Autodesk Inventor part; units mm, degrees
(part 2 of 4)
  arc A605 (9.3443, -15.2712) -> (9.707, -15.104) centre (0.9435, 3.4284) ccw
  arc A606 (10.7855, -14.5545) -> (11.1341, -14.3593) centre (0.9435, 3.4284) ccw
  arc A607 (12.1661, -13.7268) -> (12.4983, -13.5049) centre (0.9435, 3.4284) ccw
  arc A608 (13.4775, -12.7935) -> (13.7912, -12.5461) centre (0.9435, 3.4284) ccw
  arc A609 (14.7116, -11.76) -> (15.005, -11.4889) centre (0.9435, 3.4284) ccw
  arc A610 (15.8608, -10.633) -> (16.132, -10.3397) centre (0.9435, 3.4284) ccw
  arc A611 (16.9181, -9.4192) -> (17.1654, -9.1055) centre (0.9435, 3.4284) ccw
  arc A612 (17.8769, -8.1263) -> (18.0988, -7.7941) centre (0.9435, 3.4284) ccw
  arc A613 (18.7313, -6.7621) -> (18.9264, -6.4136) centre (0.9435, 3.4284) ccw
  arc A614 (19.476, -5.3351) -> (19.6432, -4.9723) centre (0.9435, 3.4284) ccw
  arc A615 (20.1064, -3.854) -> (20.2447, -3.4792) centre (0.9435, 3.4284) ccw
  arc A616 (20.6187, -2.3281) -> (20.7271, -1.9436) centre (0.9435, 3.4284) ccw
  arc A617 (21.0097, -0.7666) -> (21.0876, -0.3748) centre (0.9435, 3.4284) ccw
  arc A618 (21.277, 0.8207) -> (21.3239, 1.2174) centre (0.9435, 3.4284) ccw
  arc A619 (21.4189, 2.4241) -> (21.4346, 2.8232) centre (0.9435, 3.4284) ccw
  arc A620 (21.4346, 4.0336) -> (21.4189, 4.4328) centre (0.9435, 3.4284) ccw
  arc A621 (21.3239, 5.6395) -> (21.277, 6.0362) centre (0.9435, 3.4284) ccw
  arc A622 (21.0876, 7.2317) -> (21.0097, 7.6235) centre (0.9435, 3.4284) ccw
  arc A623 (20.7271, 8.8005) -> (20.6187, 9.1849) centre (0.9435, 3.4284) ccw
  arc A624 (20.2447, 10.3361) -> (20.1064, 10.7109) centre (0.9435, 3.4284) ccw
  arc A625 (19.6432, 11.8292) -> (19.476, 12.1919) centre (0.9435, 3.4284) ccw
  arc A626 (18.9264, 13.2704) -> (18.7313, 13.619) centre (0.9435, 3.4284) ccw
  arc A627 (18.0988, 14.651) -> (17.8769, 14.9832) centre (0.9435, 3.4284) ccw
  arc A628 (17.1654, 15.9624) -> (16.9181, 16.2761) centre (0.9435, 3.4284) ccw
  arc A629 (16.132, 17.1965) -> (15.8608, 17.4899) centre (0.9435, 3.4284) ccw
  arc A630 (15.005, 18.3458) -> (14.7116, 18.6169) centre (0.9435, 3.4284) ccw
  arc A631 (13.7912, 19.403) -> (13.4775, 19.6503) centre (0.9435, 3.4284) ccw
  arc A632 (12.4983, 20.3618) -> (12.1661, 20.5837) centre (0.9435, 3.4284) ccw
  arc A633 (11.1341, 21.2162) -> (10.7855, 21.4113) centre (0.9435, 3.4284) ccw
  arc A634 (9.707, 21.9609) -> (9.3443, 22.1281) centre (0.9435, 3.4284) ccw
  arc A635 (8.226, 22.5913) -> (7.8512, 22.7296) centre (0.9435, 3.4284) ccw
  arc A636 (6.7, 23.1036) -> (6.3156, 23.212) centre (0.9435, 3.4284) ccw
  arc A637 (5.1386, 23.4946) -> (4.7468, 23.5725) centre (0.9435, 3.4284) ccw
  arc A638 (3.5513, 23.7619) -> (3.1546, 23.8088) centre (0.9435, 3.4284) ccw
  arc A639 (1.9479, 23.9038) -> (1.5487, 23.9195) centre (0.9435, 3.4284) ccw
  line L0 (-21.5565, 3.4284) -> (23.4435, 3.4284)
  line L1 (0.9435, -19.0716) -> (0.9435, 25.9284)
  point P0 (0, 0)
  constraints: 960 point on circle, 480 centre point, 4 end point, 2 horizontal alignment, 2 vertical alignment, 476 other
extrude "押し出し1" add sketch "スケッチ1" along normal blind 3
sketch "スケッチ2" plane through (0, 0, 3) normal (0, 0, 1) x (1, 0, 0)
  arc A0 (1.2215, 23.1029) -> (1.1332, 22.8025) centre (6.2327, 21.4655) ccw projected
  arc A1 (1.1332, 22.8025) -> (0.7539, 22.8025) centre (0.9435, 3.4284) ccw projected
  arc A2 (0.7539, 22.8025) -> (0.6655, 23.1029) centre (-4.3457, 21.4655) ccw projected
  arc A3 (0.6655, 23.1029) -> (0.5317, 23.4735) centre (-5.4255, 21.1133) ccw projected
  arc A4 (0.5317, 23.4735) -> (0.3383, 23.9195) centre (-6.5223, 20.6793) ccw projected
  arc A5 (0.3383, 23.9195) -> (-0.0608, 23.9038) centre (0.9435, 3.4284) ccw projected
  arc A6 (-0.0608, 23.9038) -> (-0.2187, 23.444) centre (7.0329, 21.2118) ccw projected
  arc A7 (-0.2187, 23.444) -> (-0.323, 23.0641) centre (5.9054, 21.5585) ccw projected
  arc A8 (-0.323, 23.0641) -> (-0.3875, 22.7577) centre (4.8013, 21.8249) ccw projected
  arc A9 (-0.3875, 22.7577) -> (-0.7656, 22.7279) centre (0.9435, 3.4284) ccw projected
  arc A10 (-0.7656, 22.7279) -> (-0.8773, 23.0205) centre (-5.7445, 20.995) ccw projected
  arc A11 (-0.8773, 23.0205) -> (-1.0397, 23.3794) centre (-6.7934, 20.5591) ccw projected
  arc A12 (-1.0397, 23.3794) -> (-1.2675, 23.8088) centre (-7.8528, 20.0403) ccw projected
  arc A13 (-1.2675, 23.8088) -> (-1.6642, 23.7619) centre (0.9435, 3.4284) ccw projected
  arc A14 (-1.6642, 23.7619) -> (-1.7855, 23.2911) centre (5.6188, 21.6348) ccw projected
  arc A15 (-1.7855, 23.2911) -> (-1.8597, 22.9042) centre (4.4676, 21.8919) ccw projected
  arc A16 (-1.8597, 22.9042) -> (-1.9, 22.5936) centre (3.346, 22.0709) ccw projected
  arc A17 (-1.9, 22.5936) -> (-2.2745, 22.5343) centre (0.9435, 3.4284) ccw projected
  arc A18 (-2.2745, 22.5343) -> (-2.4088, 22.8172) centre (-7.1022, 20.4161) ccw projected
  arc A19 (-2.4088, 22.8172) -> (-2.5989, 23.1623) centre (-8.1136, 19.8993) ccw projected
  arc A20 (-2.5989, 23.1623) -> (-2.8597, 23.5725) centre (-9.129, 19.299) ccw projected
  arc A21 (-2.8597, 23.5725) -> (-3.2515, 23.4946) centre (0.9435, 3.4284) ccw projected
  arc A22 (-3.2515, 23.4946) -> (-3.3355, 23.0158) centre (4.176, 21.9455) ccw projected
  arc A23 (-3.3355, 23.0158) -> (-3.3791, 22.6242) centre (3.0081, 22.1115) ccw projected
  arc A24 (-3.3791, 22.6242) -> (-3.3949, 22.3115) centre (1.8759, 22.2019) ccw projected
  arc A25 (-3.3949, 22.3115) -> (-3.7636, 22.2229) centre (0.9435, 3.4284) ccw projected
  arc A26 (-3.7636, 22.2229) -> (-3.9197, 22.4944) centre (-8.4102, 19.7324) ccw projected
  arc A27 (-3.9197, 22.4944) -> (-4.1363, 22.8235) centre (-9.378, 19.1379) ccw projected
  arc A28 (-4.1363, 22.8235) -> (-4.4285, 23.212) centre (-10.3432, 18.4597) ccw projected
  arc A29 (-4.4285, 23.212) -> (-4.813, 23.1036) centre (0.9435, 3.4284) ccw projected
  arc A30 (-4.813, 23.1036) -> (-4.8591, 22.6197) centre (2.7132, 22.142) ccw projected
  arc A31 (-4.8591, 22.6197) -> (-4.8718, 22.2259) centre (1.5359, 22.2159) ccw projected
  arc A32 (-4.8718, 22.2259) -> (-4.863, 21.9129) centre (0.4001, 22.2172) ccw projected
  arc A33 (-4.863, 21.9129) -> (-5.2237, 21.7957) centre (0.9435, 3.4284) ccw projected
  arc A34 (-5.2237, 21.7957) -> (-5.4006, 22.0541) centre (-9.6606, 18.9483) ccw projected
  arc A35 (-5.4006, 22.0541) -> (-5.6424, 22.3652) centre (-10.5787, 18.2796) ccw projected
  arc A36 (-5.6424, 22.3652) -> (-5.9641, 22.7296) centre (-11.4877, 17.5279) ccw projected
  arc A37 (-5.9641, 22.7296) -> (-6.3389, 22.5913) centre (0.9435, 3.4284) ccw projected
  arc A38 (-6.3389, 22.5913) -> (-6.3469, 22.1053) centre (1.2395, 22.2232) ccw projected
  arc A39 (-6.3469, 22.1053) -> (-6.3287, 21.7117) centre (0.06, 22.2045) ccw projected
  arc A40 (-6.3287, 21.7117) -> (-6.2954, 21.4003) centre (-1.0724, 22.1166) ccw projected
  arc A41 (-6.2954, 21.4003) -> (-6.6458, 21.2552) centre (0.9435, 3.4284) ccw projected
  arc A42 (-6.6458, 21.2552) -> (-6.8424, 21.4989) centre (-10.8456, 18.0685) ccw projected
  arc A43 (-6.8424, 21.4989) -> (-7.1078, 21.7901) centre (-11.7084, 17.3298) ccw projected
  arc A44 (-7.1078, 21.7901) -> (-7.4572, 22.1281) centre (-12.5556, 16.5091) ccw projected
  arc A45 (-7.4572, 22.1281) -> (-7.82, 21.9609) centre (0.9435, 3.4284) ccw projected
  arc A46 (-7.82, 21.9609) -> (-7.7898, 21.4757) centre (-0.2361, 22.1885) ccw projected
  arc A47 (-7.7898, 21.4757) -> (-7.7408, 21.0848) centre (-1.4104, 22.0773) ccw projected
  arc A48 (-7.7408, 21.0848) -> (-7.6832, 20.7769) centre (-2.5324, 21.9009) ccw projected
  arc A49 (-7.6832, 20.7769) -> (-8.0211, 20.6048) centre (0.9435, 3.4284) ccw projected
  arc A50 (-8.0211, 20.6048) -> (-8.2362, 20.8323) centre (-11.9579, 17.0984) ccw projected
  arc A51 (-8.2362, 20.8323) -> (-8.5237, 21.1018) centre (-12.7601, 16.2943) ccw projected
  arc A52 (-8.5237, 21.1018) -> (-8.8985, 21.4113) centre (-13.5403, 15.4096) ccw projected
  arc A53 (-8.8985, 21.4113) -> (-9.247, 21.2162) centre (0.9435, 3.4284) ccw projected
  arc A54 (-9.247, 21.2162) -> (-9.1789, 20.7348) centre (-1.7043, 22.0381) ccw projected
  arc A55 (-9.1789, 20.7348) -> (-9.0993, 20.349) centre (-2.8663, 21.8351) ccw projected
  arc A56 (-9.0993, 20.349) -> (-9.0177, 20.0466) centre (-3.971, 21.5712) ccw projected
  arc A57 (-9.0177, 20.0466) -> (-9.3411, 19.8485) centre (0.9435, 3.4284) ccw projected
  arc A58 (-9.3411, 19.8485) -> (-9.5734, 20.0585) centre (-12.9906, 16.044) ccw projected
  arc A59 (-9.5734, 20.0585) -> (-9.8811, 20.3045) centre (-13.7273, 15.1795) ccw projected
  arc A60 (-9.8811, 20.3045) -> (-10.279, 20.5837) centre (-14.4357, 14.2363) ccw projected
  arc A61 (-10.279, 20.5837) -> (-10.6112, 20.3618) centre (0.9435, 3.4284) ccw projected
  arc A62 (-10.6112, 20.3618) -> (-10.5055, 19.8873) centre (-3.1562, 21.773) ccw projected
  arc A63 (-10.5055, 19.8873) -> (-10.3959, 19.5089) centre (-4.2988, 21.4794) ccw projected
  arc A64 (-10.3959, 19.5089) -> (-10.2909, 19.2138) centre (-5.3794, 21.1297) ccw projected
  arc A65 (-10.2909, 19.2138) -> (-10.5977, 18.9909) centre (0.9435, 3.4284) ccw projected
  arc A66 (-10.5977, 18.9909) -> (-10.8458, 19.182) centre (-13.9375, 14.9118) ccw projected
  arc A67 (-10.8458, 19.182) -> (-11.1718, 19.4032) centre (-14.604, 13.9922) ccw projected
  arc A68 (-11.1718, 19.4032) -> (-11.5904, 19.6503) centre (-15.2362, 12.9963) ccw projected
  arc A69 (-11.5904, 19.6503) -> (-11.9041, 19.403) centre (0.9435, 3.4284) ccw projected
  arc A70 (-11.9041, 19.403) -> (-11.7616, 18.9383) centre (-4.5829, 21.3947) ccw projected
  arc A71 (-11.7616, 18.9383) -> (-11.6226, 18.5696) centre (-5.6989, 21.0125) ccw projected
  arc A72 (-11.6226, 18.5696) -> (-11.4947, 18.2837) centre (-6.7487, 20.579) ccw projected
  arc A73 (-11.4947, 18.2837) -> (-11.7831, 18.0374) centre (0.9435, 3.4284) ccw projected
  arc A74 (-11.7831, 18.0374) -> (-12.0454, 18.2085) centre (-14.7926, 13.7089) ccw projected
  arc A75 (-12.0454, 18.2085) -> (-12.3878, 18.4034) centre (-15.3849, 12.7398) ccw projected
  arc A76 (-12.3878, 18.4034) -> (-12.8246, 18.6169) centre (-15.9371, 11.6974) ccw projected
  arc A77 (-12.8246, 18.6169) -> (-13.1179, 18.3458) centre (0.9435, 3.4284) ccw projected
  arc A78 (-13.1179, 18.3458) -> (-12.9393, 17.8936) centre (-5.9755, 20.9058) ccw projected
  arc A79 (-12.9393, 17.8936) -> (-12.7719, 17.537) centre (-7.058, 20.4371) ccw projected
  arc A80 (-12.7719, 17.537) -> (-12.6219, 17.2621) centre (-8.0706, 19.9226) ccw projected
  arc A81 (-12.6219, 17.2621) -> (-12.8901, 16.9939) centre (0.9435, 3.4284) ccw projected
  arc A82 (-12.8901, 16.9939) -> (-13.165, 17.1438) centre (-15.5507, 12.4426) ccw projected
  arc A83 (-13.165, 17.1438) -> (-13.5217, 17.3113) centre (-16.0652, 11.43) ccw projected
  arc A84 (-13.5217, 17.3113) -> (-13.9738, 17.4899) centre (-16.5338, 10.3475) ccw projected
  arc A85 (-13.9738, 17.4899) -> (-14.2449, 17.1965) centre (0.9435, 3.4284) ccw projected
  arc A86 (-14.2449, 17.1965) -> (-14.0314, 16.7598) centre (-7.3254, 20.309) ccw projected
  arc A87 (-14.0314, 16.7598) -> (-13.8365, 16.4174) centre (-8.3678, 19.7569) ccw projected
  arc A88 (-13.8365, 16.4174) -> (-13.6655, 16.1551) centre (-9.3369, 19.1645) ccw projected
  arc A89 (-13.6655, 16.1551) -> (-13.9118, 15.8667) centre (0.9435, 3.4284) ccw projected
  arc A90 (-13.9118, 15.8667) -> (-14.1976, 15.9946) centre (-16.2071, 11.1207) ccw projected
  arc A91 (-14.1976, 15.9946) -> (-14.5663, 16.1335) centre (-16.6405, 10.0708) ccw projected
  arc A92 (-14.5663, 16.1335) -> (-15.0311, 16.2761) centre (-17.0228, 8.9549) ccw projected
  arc A93 (-15.0311, 16.2761) -> (-15.2784, 15.9624) centre (0.9435, 3.4284) ccw projected
  arc A94 (-15.2784, 15.9624) -> (-15.0312, 15.5438) centre (-8.6244, 19.6082) ccw projected
  arc A95 (-15.0312, 15.5438) -> (-14.8101, 15.2177) centre (-9.6202, 18.976) ccw projected
  arc A96 (-14.8101, 15.2177) -> (-14.619, 14.9696) centre (-10.5399, 18.3094) ccw projected
  arc A97 (-14.619, 14.9696) -> (-14.8419, 14.6628) centre (0.9435, 3.4284) ccw projected
  arc A98 (-14.8419, 14.6628) -> (-15.1369, 14.7679) centre (-16.7577, 9.7513) ccw projected
  arc A99 (-15.1369, 14.7679) -> (-15.5153, 14.8775) centre (-17.1075, 8.6707) ccw projected
  arc A100 (-15.5153, 14.8775) -> (-15.9898, 14.9832) centre (-17.401, 7.5282) ccw projected
  arc A101 (-15.9898, 14.9832) -> (-16.2118, 14.651) centre (0.9435, 3.4284) ccw projected
  arc A102 (-16.2118, 14.651) -> (-15.9326, 14.2531) centre (-9.8643, 18.8076) ccw projected
  arc A103 (-15.9326, 14.2531) -> (-15.6865, 13.9454) centre (-10.8075, 18.0992) ccw projected
  arc A104 (-15.6865, 13.9454) -> (-15.4765, 13.713) centre (-11.672, 17.3626) ccw projected
  arc A105 (-15.4765, 13.713) -> (-15.6747, 13.3897) centre (0.9435, 3.4284) ccw projected
  arc A106 (-15.6747, 13.3897) -> (-15.977, 13.4713) centre (-17.1992, 8.343) ccw projected
  arc A107 (-15.977, 13.4713) -> (-16.3629, 13.5508) centre (-17.4631, 7.2383) ccw projected
  arc A108 (-16.3629, 13.5508) -> (-16.8442, 13.619) centre (-17.6661, 6.0763) ccw projected
  arc A109 (-16.8442, 13.619) -> (-17.0394, 13.2704) centre (0.9435, 3.4284) ccw projected
  arc A110 (-17.0394, 13.2704) -> (-16.7298, 12.8956) centre (-11.0376, 17.9123) ccw projected
  arc A111 (-16.7298, 12.8956) -> (-16.4604, 12.6082) centre (-11.9224, 17.132) ccw projected
  arc A112 (-16.4604, 12.6082) -> (-16.2328, 12.393) centre (-12.7264, 16.3298) ccw projected
  arc A113 (-16.2328, 12.393) -> (-16.405, 12.0551) centre (0.9435, 3.4284) ccw projected
  arc A114 (-16.405, 12.0551) -> (-16.7128, 12.1128) centre (-17.5289, 6.9044) ccw projected
  arc A115 (-16.7128, 12.1128) -> (-17.1037, 12.1618) centre (-17.7053, 5.7824) ccw projected
  arc A116 (-17.1037, 12.1618) -> (-17.5889, 12.1919) centre (-17.8165, 4.608) ccw projected
  arc A117 (-17.5889, 12.1919) -> (-17.7561, 11.8292) centre (0.9435, 3.4284) ccw projected
  arc A118 (-17.7561, 11.8292) -> (-17.4181, 11.4798) centre (-12.1371, 16.9276) ccw projected
  arc A119 (-17.4181, 11.4798) -> (-17.127, 11.2144) centre (-12.9579, 16.0804) ccw projected
  arc A120 (-17.127, 11.2144) -> (-16.8832, 11.0178) centre (-13.6965, 15.2175) ccw projected
  arc A121 (-16.8832, 11.0178) -> (-17.0283, 10.6674) centre (0.9435, 3.4284) ccw projected
  arc A122 (-17.0283, 10.6674) -> (-17.3397, 10.7007) centre (-17.7447, 5.4443) ccw projected
  arc A123 (-17.3397, 10.7007) -> (-17.7333, 10.7189) centre (-17.8325, 4.312) ccw projected
  arc A124 (-17.7333, 10.7189) -> (-18.2193, 10.7109) centre (-17.8512, 3.1325) ccw projected
  arc A125 (-18.2193, 10.7109) -> (-18.3576, 10.3361) centre (0.9435, 3.4284) ccw projected
  arc A126 (-18.3576, 10.3361) -> (-17.9932, 10.0143) centre (-13.1559, 15.8597) ccw projected
  arc A127 (-17.9932, 10.0143) -> (-17.6821, 9.7726) centre (-13.9077, 14.9507) ccw projected
  arc A128 (-17.6821, 9.7726) -> (-17.4237, 9.5957) centre (-14.5763, 14.0325) ccw projected
  arc A129 (-17.4237, 9.5957) -> (-17.5409, 9.235) centre (0.9435, 3.4284) ccw projected
  arc A130 (-17.5409, 9.235) -> (-17.8539, 9.2438) centre (-17.8452, 3.9719) ccw projected
  arc A131 (-17.8539, 9.2438) -> (-18.2477, 9.2311) centre (-17.8439, 2.8361) ccw projected
  arc A132 (-18.2477, 9.2311) -> (-18.7317, 9.1849) centre (-17.7701, 1.6588) ccw projected
  arc A133 (-18.7317, 9.1849) -> (-18.8401, 8.8005) centre (0.9435, 3.4284) ccw projected
  arc A134 (-18.8401, 8.8005) -> (-18.4516, 8.5083) centre (-14.0878, 14.7151) ccw projected
  arc A135 (-18.4516, 8.5083) -> (-18.1225, 8.2917) centre (-14.7659, 13.7499) ccw projected
  arc A136 (-18.1225, 8.2917) -> (-17.851, 8.1356) centre (-15.3605, 12.7822) ccw projected
  arc A137 (-17.851, 8.1356) -> (-17.9395, 7.7668) centre (0.9435, 3.4284) ccw projected
  arc A138 (-17.9395, 7.7668) -> (-18.2523, 7.751) centre (-17.8299, 2.496) ccw projected
  arc A139 (-18.2523, 7.751) -> (-18.6438, 7.7074) centre (-17.7396, 1.3639) ccw projected
  arc A140 (-18.6438, 7.7074) -> (-19.1226, 7.6235) centre (-17.5735, 0.196) ccw projected
  arc A141 (-19.1226, 7.6235) -> (-19.2006, 7.2317) centre (0.9435, 3.4284) ccw projected
  arc A142 (-19.2006, 7.2317) -> (-18.7903, 6.9709) centre (-14.927, 13.501) ccw projected
  arc A143 (-18.7903, 6.9709) -> (-18.4453, 6.7808) centre (-15.5273, 12.4856) ccw projected
  arc A144 (-18.4453, 6.7808) -> (-18.1624, 6.6465) centre (-16.0441, 11.4741) ccw projected
  arc A145 (-18.1624, 6.6465) -> (-18.2217, 6.2719) centre (0.9435, 3.4284) ccw projected
  arc A146 (-18.2217, 6.2719) -> (-18.5322, 6.2316) centre (-17.6989, 1.026) ccw projected
  arc A147 (-18.5322, 6.2316) -> (-18.9192, 6.1575) centre (-17.52, -0.0956) ccw projected
  arc A148 (-18.9192, 6.1575) -> (-19.3899, 6.0362) centre (-17.2628, -1.2469) ccw projected
  arc A149 (-19.3899, 6.0362) -> (-19.4369, 5.6395) centre (0.9435, 3.4284) ccw projected
  arc A150 (-19.4369, 5.6395) -> (-19.0075, 5.4117) centre (-15.6684, 12.2248) ccw projected
  arc A151 (-19.0075, 5.4117) -> (-18.6485, 5.2492) centre (-16.1872, 11.1654) ccw projected
  arc A152 (-18.6485, 5.2492) -> (-18.3559, 5.1375) centre (-16.623, 10.1165) ccw projected
  arc A153 (-18.3559, 5.1375) -> (-18.3857, 4.7595) centre (0.9435, 3.4284) ccw projected
  arc A154 (-18.3857, 4.7595) -> (-18.6921, 4.6949) centre (-17.453, -0.4293) ccw projected
  arc A155 (-18.6921, 4.6949) -> (-19.0721, 4.5906) centre (-17.1866, -1.5334) ccw projected
  arc A156 (-19.0721, 4.5906) -> (-19.5319, 4.4328) centre (-16.8399, -2.6609) ccw projected
  arc A157 (-19.5319, 4.4328) -> (-19.5475, 4.0336) centre (0.9435, 3.4284) ccw projected
  arc A158 (-19.5475, 4.0336) -> (-19.1016, 3.8402) centre (-16.3073, 10.8943) ccw projected
  arc A159 (-19.1016, 3.8402) -> (-18.731, 3.7064) centre (-16.7414, 9.7974) ccw projected
  arc A160 (-18.731, 3.7064) -> (-18.4305, 3.6181) centre (-17.0936, 8.7176) ccw projected
  arc A161 (-18.4305, 3.6181) -> (-18.4305, 3.2388) centre (0.9435, 3.4284) ccw projected
  arc A162 (-18.4305, 3.2388) -> (-18.731, 3.1504) centre (-17.0936, -1.8608) ccw projected
  arc A163 (-18.731, 3.1504) -> (-19.1016, 3.0166) centre (-16.7414, -2.9406) ccw projected
  arc A164 (-19.1016, 3.0166) -> (-19.5475, 2.8232) centre (-16.3073, -4.0374) ccw projected
  arc A165 (-19.5475, 2.8232) -> (-19.5319, 2.4241) centre (0.9435, 3.4284) ccw projected
  arc A166 (-19.5319, 2.4241) -> (-19.0721, 2.2662) centre (-16.8399, 9.5178) ccw projected
  arc A167 (-19.0721, 2.2662) -> (-18.6921, 2.1619) centre (-17.1866, 8.3903) ccw projected
  arc A168 (-18.6921, 2.1619) -> (-18.3857, 2.0974) centre (-17.453, 7.2862) ccw projected
  arc A169 (-18.3857, 2.0974) -> (-18.3559, 1.7193) centre (0.9435, 3.4284) ccw projected
  arc A170 (-18.3559, 1.7193) -> (-18.6485, 1.6076) centre (-16.623, -3.2596) ccw projected
  arc A171 (-18.6485, 1.6076) -> (-19.0075, 1.4452) centre (-16.1872, -4.3085) ccw projected
  arc A172 (-19.0075, 1.4452) -> (-19.4369, 1.2174) centre (-15.6684, -5.3679) ccw projected
  arc A173 (-19.4369, 1.2174) -> (-19.3899, 0.8207) centre (0.9435, 3.4284) ccw projected
  arc A174 (-19.3899, 0.8207) -> (-18.9192, 0.6994) centre (-17.2628, 8.1037) ccw projected
  arc A175 (-18.9192, 0.6994) -> (-18.5322, 0.6252) centre (-17.52, 6.9525) ccw projected
  arc A176 (-18.5322, 0.6252) -> (-18.2217, 0.585) centre (-17.6989, 5.8309) ccw projected
  arc A177 (-18.2217, 0.585) -> (-18.1624, 0.2104) centre (0.9435, 3.4284) ccw projected
  arc A178 (-18.1624, 0.2104) -> (-18.4453, 0.0761) centre (-16.0441, -4.6173) ccw projected
  arc A179 (-18.4453, 0.0761) -> (-18.7903, -0.114) centre (-15.5273, -5.6287) ccw projected
  arc A180 (-18.7903, -0.114) -> (-19.2006, -0.3748) centre (-14.927, -6.6441) ccw projected
  arc A181 (-19.2006, -0.3748) -> (-19.1226, -0.7666) centre (0.9435, 3.4284) ccw projected
  arc A182 (-19.1226, -0.7666) -> (-18.6438, -0.8506) centre (-17.5735, 6.6609) ccw projected
  arc A183 (-18.6438, -0.8506) -> (-18.2523, -0.8942) centre (-17.7396, 5.493) ccw projected
  arc A184 (-18.2523, -0.8942) -> (-17.9395, -0.91) centre (-17.8299, 4.3608) ccw projected
  arc A185 (-17.9395, -0.91) -> (-17.851, -1.2787) centre (0.9435, 3.4284) ccw projected
  arc A186 (-17.851, -1.2787) -> (-18.1225, -1.4348) centre (-15.3605, -5.9253) ccw projected
  arc A187 (-18.1225, -1.4348) -> (-18.4516, -1.6514) centre (-14.7659, -6.8931) ccw projected
  arc A188 (-18.4516, -1.6514) -> (-18.8401, -1.9436) centre (-14.0878, -7.8583) ccw projected
  arc A189 (-18.8401, -1.9436) -> (-18.7317, -2.3281) centre (0.9435, 3.4284) ccw projected
  arc A190 (-18.7317, -2.3281) -> (-18.2477, -2.3742) centre (-17.7701, 5.1981) ccw projected
  arc A191 (-18.2477, -2.3742) -> (-17.8539, -2.3869) centre (-17.8439, 4.0208) ccw projected
  arc A192 (-17.8539, -2.3869) -> (-17.5409, -2.3781) centre (-17.8452, 2.885) ccw projected
  arc A193 (-17.5409, -2.3781) -> (-17.4237, -2.7388) centre (0.9435, 3.4284) ccw projected
  arc A194 (-17.4237, -2.7388) -> (-17.6821, -2.9157) centre (-14.5763, -7.1757) ccw projected
  arc A195 (-17.6821, -2.9157) -> (-17.9932, -3.1575) centre (-13.9077, -8.0938) ccw projected
  arc A196 (-17.9932, -3.1575) -> (-18.3576, -3.4792) centre (-13.1559, -9.0028) ccw projected
  arc A197 (-18.3576, -3.4792) -> (-18.2193, -3.854) centre (0.9435, 3.4284) ccw projected
  arc A198 (-18.2193, -3.854) -> (-17.7333, -3.862) centre (-17.8512, 3.7244) ccw projected
  arc A199 (-17.7333, -3.862) -> (-17.3397, -3.8438) centre (-17.8325, 2.5449) ccw projected
  arc A200 (-17.3397, -3.8438) -> (-17.0283, -3.8105) centre (-17.7447, 1.4125) ccw projected
  arc A201 (-17.0283, -3.8105) -> (-16.8832, -4.1609) centre (0.9435, 3.4284) ccw projected
  arc A202 (-16.8832, -4.1609) -> (-17.127, -4.3575) centre (-13.6965, -8.3607) ccw projected
  arc A203 (-17.127, -4.3575) -> (-17.4181, -4.6229) centre (-12.9579, -9.2235) ccw projected
  arc A204 (-17.4181, -4.6229) -> (-17.7561, -4.9723) centre (-12.1371, -10.0707) ccw projected
  arc A205 (-17.7561, -4.9723) -> (-17.5889, -5.3351) centre (0.9435, 3.4284) ccw projected
  arc A206 (-17.5889, -5.3351) -> (-17.1037, -5.3049) centre (-17.8165, 2.2488) ccw projected
  arc A207 (-17.1037, -5.3049) -> (-16.7128, -5.2559) centre (-17.7053, 1.0745) ccw projected
  arc A208 (-16.7128, -5.2559) -> (-16.405, -5.1983) centre (-17.5289, -0.0475) ccw projected
  arc A209 (-16.405, -5.1983) -> (-16.2328, -5.5362) centre (0.9435, 3.4284) ccw projected
  arc A210 (-16.2328, -5.5362) -> (-16.4604, -5.7513) centre (-12.7264, -9.473) ccw projected
  arc A211 (-16.4604, -5.7513) -> (-16.7298, -6.0388) centre (-11.9224, -10.2752) ccw projected
  arc A212 (-16.7298, -6.0388) -> (-17.0394, -6.4136) centre (-11.0376, -11.0554) ccw projected
  arc A213 (-17.0394, -6.4136) -> (-16.8442, -6.7621) centre (0.9435, 3.4284) ccw projected
  arc A214 (-16.8442, -6.7621) -> (-16.3629, -6.694) centre (-17.6661, 0.7806) ccw projected
  arc A215 (-16.3629, -6.694) -> (-15.977, -6.6144) centre (-17.4631, -0.3814) ccw projected
  arc A216 (-15.977, -6.6144) -> (-15.6747, -6.5328) centre (-17.1992, -1.4861) ccw projected
  arc A217 (-15.6747, -6.5328) -> (-15.4765, -6.8562) centre (0.9435, 3.4284) ccw projected
  arc A218 (-15.4765, -6.8562) -> (-15.6865, -7.0885) centre (-11.672, -10.5057) ccw projected
  arc A219 (-15.6865, -7.0885) -> (-15.9326, -7.3962) centre (-10.8075, -11.2424) ccw projected
  arc A220 (-15.9326, -7.3962) -> (-16.2118, -7.7941) centre (-9.8643, -11.9508) ccw projected
  arc A221 (-16.2118, -7.7941) -> (-15.9898, -8.1263) centre (0.9435, 3.4284) ccw projected
  arc A222 (-15.9898, -8.1263) -> (-15.5153, -8.0206) centre (-17.401, -0.6713) ccw projected
  arc A223 (-15.5153, -8.0206) -> (-15.1369, -7.911) centre (-17.1075, -1.8139) ccw projected
  arc A224 (-15.1369, -7.911) -> (-14.8419, -7.8059) centre (-16.7577, -2.8945) ccw projected
  arc A225 (-14.8419, -7.8059) -> (-14.619, -8.1128) centre (0.9435, 3.4284) ccw projected
  arc A226 (-14.619, -8.1128) -> (-14.8101, -8.3609) centre (-10.5399, -11.4526) ccw projected
  arc A227 (-14.8101, -8.3609) -> (-15.0312, -8.6869) centre (-9.6202, -12.1191) ccw projected
  arc A228 (-15.0312, -8.6869) -> (-15.2784, -9.1055) centre (-8.6244, -12.7513) ccw projected
  arc A229 (-15.2784, -9.1055) -> (-15.0311, -9.4192) centre (0.9435, 3.4284) ccw projected
  arc A230 (-15.0311, -9.4192) -> (-14.5663, -9.2767) centre (-17.0228, -2.098) ccw projected
  arc A231 (-14.5663, -9.2767) -> (-14.1976, -9.1377) centre (-16.6405, -3.214) ccw projected
  arc A232 (-14.1976, -9.1377) -> (-13.9118, -9.0098) centre (-16.2071, -4.2638) ccw projected
  arc A233 (-13.9118, -9.0098) -> (-13.6655, -9.2982) centre (0.9435, 3.4284) ccw projected
  arc A234 (-13.6655, -9.2982) -> (-13.8365, -9.5605) centre (-9.3369, -12.3077) ccw projected
  arc A235 (-13.8365, -9.5605) -> (-14.0314, -9.9029) centre (-8.3678, -12.9) ccw projected
  arc A236 (-14.0314, -9.9029) -> (-14.2449, -10.3397) centre (-7.3254, -13.4522) ccw projected
  arc A237 (-14.2449, -10.3397) -> (-13.9738, -10.633) centre (0.9435, 3.4284) ccw projected
  arc A238 (-13.9738, -10.633) -> (-13.5217, -10.4544) centre (-16.5338, -3.4906) ccw projected
  arc A239 (-13.5217, -10.4544) -> (-13.165, -10.287) centre (-16.0652, -4.5731) ccw projected
  arc A240 (-13.165, -10.287) -> (-12.8901, -10.137) centre (-15.5507, -5.5857) ccw projected
  arc A241 (-12.8901, -10.137) -> (-12.6219, -10.4052) centre (0.9435, 3.4284) ccw projected
  arc A242 (-12.6219, -10.4052) -> (-12.7719, -10.6801) centre (-8.0706, -13.0658) ccw projected
  arc A243 (-12.7719, -10.6801) -> (-12.9393, -11.0368) centre (-7.058, -13.5803) ccw projected
  arc A244 (-12.9393, -11.0368) -> (-13.1179, -11.4889) centre (-5.9755, -14.0489) ccw projected
  arc A245 (-13.1179, -11.4889) -> (-12.8246, -11.76) centre (0.9435, 3.4284) ccw projected
  arc A246 (-12.8246, -11.76) -> (-12.3878, -11.5465) centre (-15.9371, -4.8405) ccw projected
  arc A247 (-12.3878, -11.5465) -> (-12.0454, -11.3516) centre (-15.3849, -5.8829) ccw projected
  arc A248 (-12.0454, -11.3516) -> (-11.7831, -11.1806) centre (-14.7926, -6.852) ccw projected
  arc A249 (-11.7831, -11.1806) -> (-11.4947, -11.4269) centre (0.9435, 3.4284) ccw projected
  arc A250 (-11.4947, -11.4269) -> (-11.6226, -11.7127) centre (-6.7487, -13.7222) ccw projected
  arc A251 (-11.6226, -11.7127) -> (-11.7616, -12.0814) centre (-5.6989, -14.1556) ccw projected
  arc A252 (-11.7616, -12.0814) -> (-11.9041, -12.5461) centre (-4.5829, -14.5379) ccw projected
  arc A253 (-11.9041, -12.5461) -> (-11.5904, -12.7935) centre (0.9435, 3.4284) ccw projected
  arc A254 (-11.5904, -12.7935) -> (-11.1718, -12.5463) centre (-15.2362, -6.1395) ccw projected
  arc A255 (-11.1718, -12.5463) -> (-10.8458, -12.3252) centre (-14.604, -7.1353) ccw projected
  arc A256 (-10.8458, -12.3252) -> (-10.5977, -12.1341) centre (-13.9375, -8.055) ccw projected
  arc A257 (-10.5977, -12.1341) -> (-10.2909, -12.357) centre (0.9435, 3.4284) ccw projected
  arc A258 (-10.2909, -12.357) -> (-10.3959, -12.652) centre (-5.3794, -14.2728) ccw projected
  arc A259 (-10.3959, -12.652) -> (-10.5055, -13.0304) centre (-4.2988, -14.6226) ccw projected
  arc A260 (-10.5055, -13.0304) -> (-10.6112, -13.5049) centre (-3.1562, -14.9161) ccw projected
  arc A261 (-10.6112, -13.5049) -> (-10.279, -13.7268) centre (0.9435, 3.4284) ccw projected
  arc A262 (-10.279, -13.7268) -> (-9.8811, -13.4476) centre (-14.4357, -7.3794) ccw projected
  arc A263 (-9.8811, -13.4476) -> (-9.5734, -13.2016) centre (-13.7273, -8.3226) ccw projected
  arc A264 (-9.5734, -13.2016) -> (-9.3411, -12.9916) centre (-12.9906, -9.1871) ccw projected
  arc A265 (-9.3411, -12.9916) -> (-9.0177, -13.1898) centre (0.9435, 3.4284) ccw projected
  arc A266 (-9.0177, -13.1898) -> (-9.0993, -13.4921) centre (-3.971, -14.7143) ccw projected
  arc A267 (-9.0993, -13.4921) -> (-9.1789, -13.878) centre (-2.8663, -14.9782) ccw projected
  arc A268 (-9.1789, -13.878) -> (-9.247, -14.3593) centre (-1.7043, -15.1812) ccw projected
  arc A269 (-9.247, -14.3593) -> (-8.8985, -14.5545) centre (0.9435, 3.4284) ccw projected
  arc A270 (-8.8985, -14.5545) -> (-8.5237, -14.2449) centre (-13.5403, -8.5527) ccw projected
  arc A271 (-8.5237, -14.2449) -> (-8.2362, -13.9755) centre (-12.7601, -9.4375) ccw projected
  arc A272 (-8.2362, -13.9755) -> (-8.0211, -13.7479) centre (-11.9579, -10.2415) ccw projected
  arc A273 (-8.0211, -13.7479) -> (-7.6832, -13.9201) centre (0.9435, 3.4284) ccw projected
  arc A274 (-7.6832, -13.9201) -> (-7.7408, -14.2279) centre (-2.5324, -15.044) ccw projected
  arc A275 (-7.7408, -14.2279) -> (-7.7898, -14.6188) centre (-1.4104, -15.2204) ccw projected
  arc A276 (-7.7898, -14.6188) -> (-7.82, -15.104) centre (-0.2361, -15.3316) ccw projected
  arc A277 (-7.82, -15.104) -> (-7.4572, -15.2712) centre (0.9435, 3.4284) ccw projected
  arc A278 (-7.4572, -15.2712) -> (-7.1078, -14.9332) centre (-12.5556, -9.6522) ccw projected
  arc A279 (-7.1078, -14.9332) -> (-6.8424, -14.6421) centre (-11.7084, -10.473) ccw projected
  arc A280 (-6.8424, -14.6421) -> (-6.6458, -14.3983) centre (-10.8456, -11.2116) ccw projected
  arc A281 (-6.6458, -14.3983) -> (-6.2954, -14.5434) centre (0.9435, 3.4284) ccw projected
  arc A282 (-6.2954, -14.5434) -> (-6.3287, -14.8548) centre (-1.0724, -15.2598) ccw projected
  arc A283 (-6.3287, -14.8548) -> (-6.3469, -15.2484) centre (0.06, -15.3476) ccw projected
  arc A284 (-6.3469, -15.2484) -> (-6.3389, -15.7344) centre (1.2395, -15.3663) ccw projected
  arc A285 (-6.3389, -15.7344) -> (-5.9641, -15.8727) centre (0.9435, 3.4284) ccw projected
  arc A286 (-5.9641, -15.8727) -> (-5.6424, -15.5083) centre (-11.4877, -10.671) ccw projected
  arc A287 (-5.6424, -15.5083) -> (-5.4006, -15.1972) centre (-10.5787, -11.4228) ccw projected
  arc A288 (-5.4006, -15.1972) -> (-5.2237, -14.9388) centre (-9.6606, -12.0914) ccw projected
  arc A289 (-5.2237, -14.9388) -> (-4.863, -15.056) centre (0.9435, 3.4284) ccw projected
  arc A290 (-4.863, -15.056) -> (-4.8718, -15.369) centre (0.4001, -15.3603) ccw projected
  arc A291 (-4.8718, -15.369) -> (-4.8591, -15.7628) centre (1.5359, -15.359) ccw projected
  arc A292 (-4.8591, -15.7628) -> (-4.813, -16.2467) centre (2.7132, -15.2851) ccw projected
  arc A293 (-4.813, -16.2467) -> (-4.4285, -16.3552) centre (0.9435, 3.4284) ccw projected
  arc A294 (-4.4285, -16.3552) -> (-4.1363, -15.9667) centre (-10.3432, -11.6029) ccw projected
  arc A295 (-4.1363, -15.9667) -> (-3.9197, -15.6376) centre (-9.378, -12.281) ccw projected
  arc A296 (-3.9197, -15.6376) -> (-3.7636, -15.3661) centre (-8.4102, -12.8756) ccw projected
  arc A297 (-3.7636, -15.3661) -> (-3.3949, -15.4546) centre (0.9435, 3.4284) ccw projected
  arc A298 (-3.3949, -15.4546) -> (-3.3791, -15.7674) centre (1.8759, -15.345) ccw projected
  arc A299 (-3.3791, -15.7674) -> (-3.3355, -16.1589) centre (3.0081, -15.2547) ccw projected
  arc A300 (-3.3355, -16.1589) -> (-3.2515, -16.6377) centre (4.176, -15.0886) ccw projected
  arc A301 (-3.2515, -16.6377) -> (-2.8597, -16.7157) centre (0.9435, 3.4284) ccw projected
  arc A302 (-2.8597, -16.7157) -> (-2.5989, -16.3054) centre (-9.129, -12.4421) ccw projected
  arc A303 (-2.5989, -16.3054) -> (-2.4088, -15.9604) centre (-8.1136, -13.0424) ccw projected
  arc A304 (-2.4088, -15.9604) -> (-2.2745, -15.6774) centre (-7.1022, -13.5592) ccw projected
  arc A305 (-2.2745, -15.6774) -> (-1.9, -15.7368) centre (0.9435, 3.4284) ccw projected
  arc A306 (-1.9, -15.7368) -> (-1.8597, -16.0473) centre (3.346, -15.214) ccw projected
  arc A307 (-1.8597, -16.0473) -> (-1.7855, -16.4343) centre (4.4676, -15.0351) ccw projected
  arc A308 (-1.7855, -16.4343) -> (-1.6642, -16.905) centre (5.6188, -14.7779) ccw projected
  arc A309 (-1.6642, -16.905) -> (-1.2675, -16.952) centre (0.9435, 3.4284) ccw projected
  arc A310 (-1.2675, -16.952) -> (-1.0397, -16.5225) centre (-7.8528, -13.1834) ccw projected
  arc A311 (-1.0397, -16.5225) -> (-0.8773, -16.1636) centre (-6.7934, -13.7022) ccw projected
  arc A312 (-0.8773, -16.1636) -> (-0.7656, -15.871) centre (-5.7445, -14.1381) ccw projected
  arc A313 (-0.7656, -15.871) -> (-0.3875, -15.9008) centre (0.9435, 3.4284) ccw projected
  arc A314 (-0.3875, -15.9008) -> (-0.323, -16.2072) centre (4.8013, -14.9681) ccw projected
  arc A315 (-0.323, -16.2072) -> (-0.2187, -16.5872) centre (5.9054, -14.7017) ccw projected
  arc A316 (-0.2187, -16.5872) -> (-0.0608, -17.0469) centre (7.0329, -14.355) ccw projected
  arc A317 (-0.0608, -17.0469) -> (0.3383, -17.0626) centre (0.9435, 3.4284) ccw projected
  arc A318 (0.3383, -17.0626) -> (0.5317, -16.6166) centre (-6.5223, -13.8224) ccw projected
  arc A319 (0.5317, -16.6166) -> (0.6655, -16.2461) centre (-5.4255, -14.2565) ccw projected
  arc A320 (0.6655, -16.2461) -> (0.7539, -15.9456) centre (-4.3457, -14.6087) ccw projected
  arc A321 (0.7539, -15.9456) -> (1.1332, -15.9456) centre (0.9435, 3.4284) ccw projected
  arc A322 (1.1332, -15.9456) -> (1.2215, -16.2461) centre (6.2327, -14.6087) ccw projected
  arc A323 (1.2215, -16.2461) -> (1.3553, -16.6166) centre (7.3125, -14.2565) ccw projected
  arc A324 (1.3553, -16.6166) -> (1.5487, -17.0626) centre (8.4094, -13.8224) ccw projected
  arc A325 (1.5487, -17.0626) -> (1.9479, -17.0469) centre (0.9435, 3.4284) ccw projected
  arc A326 (1.9479, -17.0469) -> (2.1057, -16.5872) centre (-5.1458, -14.355) ccw projected
  arc A327 (2.1057, -16.5872) -> (2.21, -16.2072) centre (-4.0183, -14.7017) ccw projected
  arc A328 (2.21, -16.2072) -> (2.2746, -15.9008) centre (-2.9142, -14.9681) ccw projected
  arc A329 (2.2746, -15.9008) -> (2.6526, -15.871) centre (0.9435, 3.4284) ccw projected
  arc A330 (2.6526, -15.871) -> (2.7643, -16.1636) centre (7.6316, -14.1381) ccw projected
  arc A331 (2.7643, -16.1636) -> (2.9268, -16.5225) centre (8.6805, -13.7022) ccw projected
  arc A332 (2.9268, -16.5225) -> (3.1546, -16.952) centre (9.7398, -13.1834) ccw projected
  arc A333 (3.1546, -16.952) -> (3.5513, -16.905) centre (0.9435, 3.4284) ccw projected
  arc A334 (3.5513, -16.905) -> (3.6725, -16.4343) centre (-3.7318, -14.7779) ccw projected
  arc A335 (3.6725, -16.4343) -> (3.7467, -16.0473) centre (-2.5805, -15.0351) ccw projected
  arc A336 (3.7467, -16.0473) -> (3.787, -15.7368) centre (-1.4589, -15.214) ccw projected
  arc A337 (3.787, -15.7368) -> (4.1616, -15.6774) centre (0.9435, 3.4284) ccw projected
  arc A338 (4.1616, -15.6774) -> (4.2959, -15.9604) centre (8.9892, -13.5592) ccw projected
  arc A339 (4.2959, -15.9604) -> (4.486, -16.3054) centre (10.0007, -13.0424) ccw projected
  arc A340 (4.486, -16.3054) -> (4.7468, -16.7157) centre (11.0161, -12.4421) ccw projected
  arc A341 (4.7468, -16.7157) -> (5.1386, -16.6377) centre (0.9435, 3.4284) ccw projected
  arc A342 (5.1386, -16.6377) -> (5.2225, -16.1589) centre (-2.2889, -15.0886) ccw projected
  arc A343 (5.2225, -16.1589) -> (5.2661, -15.7674) centre (-1.121, -15.2547) ccw projected
  arc A344 (5.2661, -15.7674) -> (5.2819, -15.4546) centre (0.0111, -15.345) ccw projected
  arc A345 (5.2819, -15.4546) -> (5.6507, -15.3661) centre (0.9435, 3.4284) ccw projected
  arc A346 (5.6507, -15.3661) -> (5.8068, -15.6376) centre (10.2973, -12.8756) ccw projected
  arc A347 (5.8068, -15.6376) -> (6.0234, -15.9667) centre (11.265, -12.281) ccw projected
  arc A348 (6.0234, -15.9667) -> (6.3156, -16.3552) centre (12.2302, -11.6029) ccw projected
  arc A349 (6.3156, -16.3552) -> (6.7, -16.2467) centre (0.9435, 3.4284) ccw projected
  arc A350 (6.7, -16.2467) -> (6.7462, -15.7628) centre (-0.8261, -15.2851) ccw projected
  arc A351 (6.7462, -15.7628) -> (6.7589, -15.369) centre (0.3512, -15.359) ccw projected
  arc A352 (6.7589, -15.369) -> (6.7501, -15.056) centre (1.487, -15.3603) ccw projected
  arc A353 (6.7501, -15.056) -> (7.1108, -14.9388) centre (0.9435, 3.4284) ccw projected
  arc A354 (7.1108, -14.9388) -> (7.2877, -15.1972) centre (11.5476, -12.0914) ccw projected
  arc A355 (7.2877, -15.1972) -> (7.5294, -15.5083) centre (12.4658, -11.4228) ccw projected
  arc A356 (7.5294, -15.5083) -> (7.8512, -15.8727) centre (13.3748, -10.671) ccw projected
  arc A357 (7.8512, -15.8727) -> (8.226, -15.7344) centre (0.9435, 3.4284) ccw projected
  arc A358 (8.226, -15.7344) -> (8.234, -15.2484) centre (0.6476, -15.3663) ccw projected
  arc A359 (8.234, -15.2484) -> (8.2158, -14.8548) centre (1.827, -15.3476) ccw projected
  arc A360 (8.2158, -14.8548) -> (8.1825, -14.5434) centre (2.9594, -15.2598) ccw projected
  arc A361 (8.1825, -14.5434) -> (8.5329, -14.3983) centre (0.9435, 3.4284) ccw projected
  arc A362 (8.5329, -14.3983) -> (8.7295, -14.6421) centre (12.7326, -11.2116) ccw projected
  arc A363 (8.7295, -14.6421) -> (8.9949, -14.9332) centre (13.5955, -10.473) ccw projected
  arc A364 (8.9949, -14.9332) -> (9.3443, -15.2712) centre (14.4427, -9.6522) ccw projected
  arc A365 (9.3443, -15.2712) -> (9.707, -15.104) centre (0.9435, 3.4284) ccw projected
  arc A366 (9.707, -15.104) -> (9.6769, -14.6188) centre (2.1231, -15.3316) ccw projected
  arc A367 (9.6769, -14.6188) -> (9.6279, -14.2279) centre (3.2975, -15.2204) ccw projected
  arc A368 (9.6279, -14.2279) -> (9.5702, -13.9201) centre (4.4195, -15.044) ccw projected
  arc A369 (9.5702, -13.9201) -> (9.9081, -13.7479) centre (0.9435, 3.4284) ccw projected
  arc A370 (9.9081, -13.7479) -> (10.1233, -13.9755) centre (13.8449, -10.2415) ccw projected
  arc A371 (10.1233, -13.9755) -> (10.4107, -14.2449) centre (14.6471, -9.4375) ccw projected
  arc A372 (10.4107, -14.2449) -> (10.7855, -14.5545) centre (15.4274, -8.5527) ccw projected
  arc A373 (10.7855, -14.5545) -> (11.1341, -14.3593) centre (0.9435, 3.4284) ccw projected
  arc A374 (11.1341, -14.3593) -> (11.0659, -13.878) centre (3.5914, -15.1812) ccw projected
  arc A375 (11.0659, -13.878) -> (10.9864, -13.4921) centre (4.7534, -14.9782) ccw projected
  arc A376 (10.9864, -13.4921) -> (10.9048, -13.1898) centre (5.8581, -14.7143) ccw projected
  arc A377 (10.9048, -13.1898) -> (11.2281, -12.9916) centre (0.9435, 3.4284) ccw projected
  arc A378 (11.2281, -12.9916) -> (11.4605, -13.2016) centre (14.8777, -9.1871) ccw projected
  arc A379 (11.4605, -13.2016) -> (11.7682, -13.4476) centre (15.6143, -8.3226) ccw projected
  arc A380 (11.7682, -13.4476) -> (12.1661, -13.7268) centre (16.3227, -7.3794) ccw projected
  arc A381 (12.1661, -13.7268) -> (12.4983, -13.5049) centre (0.9435, 3.4284) ccw projected
  arc A382 (12.4983, -13.5049) -> (12.3926, -13.0304) centre (5.0433, -14.9161) ccw projected
  arc A383 (12.3926, -13.0304) -> (12.283, -12.652) centre (6.1858, -14.6226) ccw projected
  arc A384 (12.283, -12.652) -> (12.1779, -12.357) centre (7.2664, -14.2728) ccw projected
  arc A385 (12.1779, -12.357) -> (12.4847, -12.1341) centre (0.9435, 3.4284) ccw projected
  arc A386 (12.4847, -12.1341) -> (12.7328, -12.3252) centre (15.8245, -8.055) ccw projected
  arc A387 (12.7328, -12.3252) -> (13.0589, -12.5463) centre (16.4911, -7.1353) ccw projected
  arc A388 (13.0589, -12.5463) -> (13.4775, -12.7935) centre (17.1233, -6.1395) ccw projected
  arc A389 (13.4775, -12.7935) -> (13.7912, -12.5461) centre (0.9435, 3.4284) ccw projected
  arc A390 (13.7912, -12.5461) -> (13.6486, -12.0814) centre (6.47, -14.5379) ccw projected
  arc A391 (13.6486, -12.0814) -> (13.5097, -11.7127) centre (7.5859, -14.1556) ccw projected
  arc A392 (13.5097, -11.7127) -> (13.3818, -11.4269) centre (8.6357, -13.7222) ccw projected
  arc A393 (13.3818, -11.4269) -> (13.6702, -11.1806) centre (0.9435, 3.4284) ccw projected
  arc A394 (13.6702, -11.1806) -> (13.9325, -11.3516) centre (16.6796, -6.852) ccw projected
  arc A395 (13.9325, -11.3516) -> (14.2749, -11.5465) centre (17.272, -5.8829) ccw projected
  arc A396 (14.2749, -11.5465) -> (14.7116, -11.76) centre (17.8241, -4.8405) ccw projected
  arc A397 (14.7116, -11.76) -> (15.005, -11.4889) centre (0.9435, 3.4284) ccw projected
  arc A398 (15.005, -11.4889) -> (14.8264, -11.0368) centre (7.8625, -14.0489) ccw projected
  arc A399 (14.8264, -11.0368) -> (14.6589, -10.6801) centre (8.9451, -13.5803) ccw projected
  arc A400 (14.6589, -10.6801) -> (14.509, -10.4052) centre (9.9577, -13.0658) ccw projected
  arc A401 (14.509, -10.4052) -> (14.7772, -10.137) centre (0.9435, 3.4284) ccw projected
  arc A402 (14.7772, -10.137) -> (15.0521, -10.287) centre (17.4377, -5.5857) ccw projected
  arc A403 (15.0521, -10.287) -> (15.4087, -10.4544) centre (17.9522, -4.5731) ccw projected
  arc A404 (15.4087, -10.4544) -> (15.8608, -10.633) centre (18.4209, -3.4906) ccw projected
  arc A405 (15.8608, -10.633) -> (16.132, -10.3397) centre (0.9435, 3.4284) ccw projected
  arc A406 (16.132, -10.3397) -> (15.9185, -9.9029) centre (9.2125, -13.4522) ccw projected
  arc A407 (15.9185, -9.9029) -> (15.7236, -9.5605) centre (10.2549, -12.9) ccw projected
  arc A408 (15.7236, -9.5605) -> (15.5525, -9.2982) centre (11.224, -12.3077) ccw projected
  arc A409 (15.5525, -9.2982) -> (15.7988, -9.0098) centre (0.9435, 3.4284) ccw projected
  arc A410 (15.7988, -9.0098) -> (16.0847, -9.1377) centre (18.0941, -4.2638) ccw projected
  arc A411 (16.0847, -9.1377) -> (16.4534, -9.2767) centre (18.5276, -3.214) ccw projected
  arc A412 (16.4534, -9.2767) -> (16.9181, -9.4192) centre (18.9098, -2.098) ccw projected
  arc A413 (16.9181, -9.4192) -> (17.1654, -9.1055) centre (0.9435, 3.4284) ccw projected
  arc A414 (17.1654, -9.1055) -> (16.9183, -8.6869) centre (10.5114, -12.7513) ccw projected
  arc A415 (16.9183, -8.6869) -> (16.6971, -8.3609) centre (11.5073, -12.1191) ccw projected
  arc A416 (16.6971, -8.3609) -> (16.506, -8.1128) centre (12.4269, -11.4526) ccw projected
  arc A417 (16.506, -8.1128) -> (16.7289, -7.8059) centre (0.9435, 3.4284) ccw projected
  arc A418 (16.7289, -7.8059) -> (17.024, -7.911) centre (18.6448, -2.8945) ccw projected
  arc A419 (17.024, -7.911) -> (17.4024, -8.0206) centre (18.9945, -1.8139) ccw projected
  arc A420 (17.4024, -8.0206) -> (17.8769, -8.1263) centre (19.2881, -0.6713) ccw projected
  arc A421 (17.8769, -8.1263) -> (18.0988, -7.7941) centre (0.9435, 3.4284) ccw projected
  arc A422 (18.0988, -7.7941) -> (17.8196, -7.3962) centre (11.7514, -11.9508) ccw projected
  arc A423 (17.8196, -7.3962) -> (17.5735, -7.0885) centre (12.6946, -11.2424) ccw projected
  arc A424 (17.5735, -7.0885) -> (17.3636, -6.8562) centre (13.5591, -10.5057) ccw projected
  arc A425 (17.3636, -6.8562) -> (17.5617, -6.5328) centre (0.9435, 3.4284) ccw projected
  arc A426 (17.5617, -6.5328) -> (17.8641, -6.6144) centre (19.0863, -1.4861) ccw projected
  arc A427 (17.8641, -6.6144) -> (18.2499, -6.694) centre (19.3502, -0.3814) ccw projected
  arc A428 (18.2499, -6.694) -> (18.7313, -6.7621) centre (19.5532, 0.7806) ccw projected
  arc A429 (18.7313, -6.7621) -> (18.9264, -6.4136) centre (0.9435, 3.4284) ccw projected
  arc A430 (18.9264, -6.4136) -> (18.6169, -6.0388) centre (12.9247, -11.0554) ccw projected
  arc A431 (18.6169, -6.0388) -> (18.3474, -5.7513) centre (13.8094, -10.2752) ccw projected
  arc A432 (18.3474, -5.7513) -> (18.1199, -5.5362) centre (14.6135, -9.473) ccw projected
  arc A433 (18.1199, -5.5362) -> (18.292, -5.1983) centre (0.9435, 3.4284) ccw projected
  arc A434 (18.292, -5.1983) -> (18.5999, -5.2559) centre (19.416, -0.0475) ccw projected
  arc A435 (18.5999, -5.2559) -> (18.9908, -5.3049) centre (19.5924, 1.0745) ccw projected
  arc A436 (18.9908, -5.3049) -> (19.476, -5.3351) centre (19.7035, 2.2488) ccw projected
  arc A437 (19.476, -5.3351) -> (19.6432, -4.9723) centre (0.9435, 3.4284) ccw projected
  arc A438 (19.6432, -4.9723) -> (19.3052, -4.6229) centre (14.0242, -10.0707) ccw projected
  arc A439 (19.3052, -4.6229) -> (19.014, -4.3575) centre (14.8449, -9.2235) ccw projected
  arc A440 (19.014, -4.3575) -> (18.7703, -4.1609) centre (15.5835, -8.3607) ccw projected
  arc A441 (18.7703, -4.1609) -> (18.9154, -3.8105) centre (0.9435, 3.4284) ccw projected
  arc A442 (18.9154, -3.8105) -> (19.2268, -3.8438) centre (19.6317, 1.4125) ccw projected
  arc A443 (19.2268, -3.8438) -> (19.6204, -3.862) centre (19.7196, 2.5449) ccw projected
  arc A444 (19.6204, -3.862) -> (20.1064, -3.854) centre (19.7383, 3.7244) ccw projected
  arc A445 (20.1064, -3.854) -> (20.2447, -3.4792) centre (0.9435, 3.4284) ccw projected
  arc A446 (20.2447, -3.4792) -> (19.8803, -3.1575) centre (15.043, -9.0028) ccw projected
  arc A447 (19.8803, -3.1575) -> (19.5692, -2.9157) centre (15.7947, -8.0938) ccw projected
  arc A448 (19.5692, -2.9157) -> (19.3108, -2.7388) centre (16.4634, -7.1757) ccw projected
  arc A449 (19.3108, -2.7388) -> (19.428, -2.3781) centre (0.9435, 3.4284) ccw projected
  arc A450 (19.428, -2.3781) -> (19.741, -2.3869) centre (19.7323, 2.885) ccw projected
  arc A451 (19.741, -2.3869) -> (20.1348, -2.3742) centre (19.731, 4.0208) ccw projected
  arc A452 (20.1348, -2.3742) -> (20.6187, -2.3281) centre (19.6571, 5.1981) ccw projected
  arc A453 (20.6187, -2.3281) -> (20.7271, -1.9436) centre (0.9435, 3.4284) ccw projected
  arc A454 (20.7271, -1.9436) -> (20.3386, -1.6514) centre (15.9748, -7.8583) ccw projected
  arc A455 (20.3386, -1.6514) -> (20.0095, -1.4348) centre (16.653, -6.8931) ccw projected
  arc A456 (20.0095, -1.4348) -> (19.738, -1.2787) centre (17.2475, -5.9253) ccw projected
  arc A457 (19.738, -1.2787) -> (19.8266, -0.91) centre (0.9435, 3.4284) ccw projected
  arc A458 (19.8266, -0.91) -> (20.1393, -0.8942) centre (19.717, 4.3608) ccw projected
  arc A459 (20.1393, -0.8942) -> (20.5309, -0.8506) centre (19.6266, 5.493) ccw projected
  arc A460 (20.5309, -0.8506) -> (21.0097, -0.7666) centre (19.4606, 6.6609) ccw projected
  arc A461 (21.0097, -0.7666) -> (21.0876, -0.3748) centre (0.9435, 3.4284) ccw projected
  arc A462 (21.0876, -0.3748) -> (20.6774, -0.114) centre (16.814, -6.6441) ccw projected
  arc A463 (20.6774, -0.114) -> (20.3323, 0.0761) centre (17.4144, -5.6287) ccw projected
  arc A464 (20.3323, 0.0761) -> (20.0494, 0.2104) centre (17.9312, -4.6173) ccw projected
  arc A465 (20.0494, 0.2104) -> (20.1087, 0.585) centre (0.9435, 3.4284) ccw projected
  arc A466 (20.1087, 0.585) -> (20.4193, 0.6252) centre (19.586, 5.8309) ccw projected
  arc A467 (20.4193, 0.6252) -> (20.8062, 0.6994) centre (19.407, 6.9525) ccw projected
  arc A468 (20.8062, 0.6994) -> (21.277, 0.8207) centre (19.1499, 8.1037) ccw projected
  arc A469 (21.277, 0.8207) -> (21.3239, 1.2174) centre (0.9435, 3.4284) ccw projected
  arc A470 (21.3239, 1.2174) -> (20.8945, 1.4452) centre (17.5554, -5.3679) ccw projected
  arc A471 (20.8945, 1.4452) -> (20.5356, 1.6076) centre (18.0742, -4.3085) ccw projected
  arc A472 (20.5356, 1.6076) -> (20.243, 1.7193) centre (18.51, -3.2596) ccw projected
  arc A473 (20.243, 1.7193) -> (20.2728, 2.0974) centre (0.9435, 3.4284) ccw projected
  arc A474 (20.2728, 2.0974) -> (20.5792, 2.1619) centre (19.34, 7.2862) ccw projected
  arc A475 (20.5792, 2.1619) -> (20.9591, 2.2662) centre (19.0736, 8.3903) ccw projected
  arc A476 (20.9591, 2.2662) -> (21.4189, 2.4241) centre (18.7269, 9.5178) ccw projected
  arc A477 (21.4189, 2.4241) -> (21.4346, 2.8232) centre (0.9435, 3.4284) ccw projected
  arc A478 (21.4346, 2.8232) -> (20.9886, 3.0166) centre (18.1944, -4.0374) ccw projected
  arc A479 (20.9886, 3.0166) -> (20.618, 3.1504) centre (18.6284, -2.9406) ccw projected
  arc A480 (20.618, 3.1504) -> (20.3176, 3.2388) centre (18.9806, -1.8608) ccw projected
  arc A481 (20.3176, 3.2388) -> (20.3176, 3.6181) centre (0.9435, 3.4284) ccw projected
  arc A482 (20.3176, 3.6181) -> (20.618, 3.7064) centre (18.9806, 8.7176) ccw projected
  arc A483 (20.618, 3.7064) -> (20.9886, 3.8402) centre (18.6284, 9.7974) ccw projected
  arc A484 (20.9886, 3.8402) -> (21.4346, 4.0336) centre (18.1944, 10.8943) ccw projected
  arc A485 (21.4346, 4.0336) -> (21.4189, 4.4328) centre (0.9435, 3.4284) ccw projected
  arc A486 (21.4189, 4.4328) -> (20.9591, 4.5906) centre (18.7269, -2.6609) ccw projected
  arc A487 (20.9591, 4.5906) -> (20.5792, 4.6949) centre (19.0736, -1.5334) ccw projected
  arc A488 (20.5792, 4.6949) -> (20.2728, 4.7595) centre (19.34, -0.4293) ccw projected
  arc A489 (20.2728, 4.7595) -> (20.243, 5.1375) centre (0.9435, 3.4284) ccw projected
  arc A490 (20.243, 5.1375) -> (20.5356, 5.2492) centre (18.51, 10.1165) ccw projected
  arc A491 (20.5356, 5.2492) -> (20.8945, 5.4117) centre (18.0742, 11.1654) ccw projected
  arc A492 (20.8945, 5.4117) -> (21.3239, 5.6395) centre (17.5554, 12.2248) ccw projected
  arc A493 (21.3239, 5.6395) -> (21.277, 6.0362) centre (0.9435, 3.4284) ccw projected
  arc A494 (21.277, 6.0362) -> (20.8062, 6.1575) centre (19.1499, -1.2469) ccw projected
  arc A495 (20.8062, 6.1575) -> (20.4193, 6.2316) centre (19.407, -0.0956) ccw projected
  arc A496 (20.4193, 6.2316) -> (20.1087, 6.2719) centre (19.586, 1.026) ccw projected
  arc A497 (20.1087, 6.2719) -> (20.0494, 6.6465) centre (0.9435, 3.4284) ccw projected
  arc A498 (20.0494, 6.6465) -> (20.3323, 6.7808) centre (17.9312, 11.4741) ccw projected
  arc A499 (20.3323, 6.7808) -> (20.6774, 6.9709) centre (17.4144, 12.4856) ccw projected
  arc A500 (20.6774, 6.9709) -> (21.0876, 7.2317) centre (16.814, 13.501) ccw projected
  arc A501 (21.0876, 7.2317) -> (21.0097, 7.6235) centre (0.9435, 3.4284) ccw projected
  arc A502 (21.0097, 7.6235) -> (20.5309, 7.7074) centre (19.4606, 0.196) ccw projected
  arc A503 (20.5309, 7.7074) -> (20.1393, 7.751) centre (19.6266, 1.3639) ccw projected
  arc A504 (20.1393, 7.751) -> (19.8266, 7.7668) centre (19.717, 2.496) ccw projected
  arc A505 (19.8266, 7.7668) -> (19.738, 8.1356) centre (0.9435, 3.4284) ccw projected
  arc A506 (19.738, 8.1356) -> (20.0095, 8.2917) centre (17.2475, 12.7822) ccw projected
  arc A507 (20.0095, 8.2917) -> (20.3386, 8.5083) centre (16.653, 13.7499) ccw projected
  arc A508 (20.3386, 8.5083) -> (20.7271, 8.8005) centre (15.9748, 14.7151) ccw projected
  arc A509 (20.7271, 8.8005) -> (20.6187, 9.1849) centre (0.9435, 3.4284) ccw projected
  arc A510 (20.6187, 9.1849) -> (20.1348, 9.2311) centre (19.6571, 1.6588) ccw projected
  arc A511 (20.1348, 9.2311) -> (19.741, 9.2438) centre (19.731, 2.8361) ccw projected
  arc A512 (19.741, 9.2438) -> (19.428, 9.235) centre (19.7323, 3.9719) ccw projected
  arc A513 (19.428, 9.235) -> (19.3108, 9.5957) centre (0.9435, 3.4284) ccw projected
  arc A514 (19.3108, 9.5957) -> (19.5692, 9.7726) centre (16.4634, 14.0325) ccw projected
  arc A515 (19.5692, 9.7726) -> (19.8803, 10.0143) centre (15.7947, 14.9507) ccw projected
  arc A516 (19.8803, 10.0143) -> (20.2447, 10.3361) centre (15.043, 15.8597) ccw projected
  arc A517 (20.2447, 10.3361) -> (20.1064, 10.7109) centre (0.9435, 3.4284) ccw projected
  arc A518 (20.1064, 10.7109) -> (19.6204, 10.7189) centre (19.7383, 3.1325) ccw projected
  arc A519 (19.6204, 10.7189) -> (19.2268, 10.7007) centre (19.7196, 4.312) ccw projected
  arc A520 (19.2268, 10.7007) -> (18.9154, 10.6674) centre (19.6317, 5.4443) ccw projected
  arc A521 (18.9154, 10.6674) -> (18.7703, 11.0178) centre (0.9435, 3.4284) ccw projected
  arc A522 (18.7703, 11.0178) -> (19.014, 11.2144) centre (15.5835, 15.2175) ccw projected
  arc A523 (19.014, 11.2144) -> (19.3052, 11.4798) centre (14.8449, 16.0804) ccw projected
  arc A524 (19.3052, 11.4798) -> (19.6432, 11.8292) centre (14.0242, 16.9276) ccw projected
  arc A525 (19.6432, 11.8292) -> (19.476, 12.1919) centre (0.9435, 3.4284) ccw projected
  arc A526 (19.476, 12.1919) -> (18.9908, 12.1618) centre (19.7035, 4.608) ccw projected
  arc A527 (18.9908, 12.1618) -> (18.5999, 12.1128) centre (19.5924, 5.7824) ccw projected
  arc A528 (18.5999, 12.1128) -> (18.292, 12.0551) centre (19.416, 6.9044) ccw projected
  arc A529 (18.292, 12.0551) -> (18.1199, 12.393) centre (0.9435, 3.4284) ccw projected
  arc A530 (18.1199, 12.393) -> (18.3474, 12.6082) centre (14.6135, 16.3298) ccw projected
  arc A531 (18.3474, 12.6082) -> (18.6169, 12.8956) centre (13.8094, 17.132) ccw projected
  arc A532 (18.6169, 12.8956) -> (18.9264, 13.2704) centre (12.9247, 17.9123) ccw projected
  arc A533 (18.9264, 13.2704) -> (18.7313, 13.619) centre (0.9435, 3.4284) ccw projected
  arc A534 (18.7313, 13.619) -> (18.2499, 13.5508) centre (19.5532, 6.0763) ccw projected
  arc A535 (18.2499, 13.5508) -> (17.8641, 13.4713) centre (19.3502, 7.2383) ccw projected
  arc A536 (17.8641, 13.4713) -> (17.5617, 13.3897) centre (19.0863, 8.343) ccw projected
  arc A537 (17.5617, 13.3897) -> (17.3636, 13.713) centre (0.9435, 3.4284) ccw projected
  arc A538 (17.3636, 13.713) -> (17.5735, 13.9454) centre (13.5591, 17.3626) ccw projected
  arc A539 (17.5735, 13.9454) -> (17.8196, 14.2531) centre (12.6946, 18.0992) ccw projected
  arc A540 (17.8196, 14.2531) -> (18.0988, 14.651) centre (11.7514, 18.8076) ccw projected
  arc A541 (18.0988, 14.651) -> (17.8769, 14.9832) centre (0.9435, 3.4284) ccw projected
  arc A542 (17.8769, 14.9832) -> (17.4024, 14.8775) centre (19.2881, 7.5282) ccw projected
  arc A543 (17.4024, 14.8775) -> (17.024, 14.7679) centre (18.9945, 8.6707) ccw projected
  arc A544 (17.024, 14.7679) -> (16.7289, 14.6628) centre (18.6448, 9.7513) ccw projected
  arc A545 (16.7289, 14.6628) -> (16.506, 14.9696) centre (0.9435, 3.4284) ccw projected
  arc A546 (16.506, 14.9696) -> (16.6971, 15.2177) centre (12.4269, 18.3094) ccw projected
  arc A547 (16.6971, 15.2177) -> (16.9183, 15.5438) centre (11.5073, 18.976) ccw projected
  arc A548 (16.9183, 15.5438) -> (17.1654, 15.9624) centre (10.5114, 19.6082) ccw projected
  arc A549 (17.1654, 15.9624) -> (16.9181, 16.2761) centre (0.9435, 3.4284) ccw projected
  arc A550 (16.9181, 16.2761) -> (16.4534, 16.1335) centre (18.9098, 8.9549) ccw projected
  arc A551 (16.4534, 16.1335) -> (16.0847, 15.9946) centre (18.5276, 10.0708) ccw projected
  arc A552 (16.0847, 15.9946) -> (15.7988, 15.8667) centre (18.0941, 11.1207) ccw projected
  arc A553 (15.7988, 15.8667) -> (15.5525, 16.1551) centre (0.9435, 3.4284) ccw projected
  arc A554 (15.5525, 16.1551) -> (15.7236, 16.4174) centre (11.224, 19.1645) ccw projected
  arc A555 (15.7236, 16.4174) -> (15.9185, 16.7598) centre (10.2549, 19.7569) ccw projected
  arc A556 (15.9185, 16.7598) -> (16.132, 17.1965) centre (9.2125, 20.309) ccw projected
  arc A557 (16.132, 17.1965) -> (15.8608, 17.4899) centre (0.9435, 3.4284) ccw projected
  arc A558 (15.8608, 17.4899) -> (15.4087, 17.3113) centre (18.4209, 10.3475) ccw projected
  arc A559 (15.4087, 17.3113) -> (15.0521, 17.1438) centre (17.9522, 11.43) ccw projected
  arc A560 (15.0521, 17.1438) -> (14.7772, 16.9939) centre (17.4377, 12.4426) ccw projected
  arc A561 (14.7772, 16.9939) -> (14.509, 17.2621) centre (0.9435, 3.4284) ccw projected
  arc A562 (14.509, 17.2621) -> (14.6589, 17.537) centre (9.9577, 19.9226) ccw projected
  arc A563 (14.6589, 17.537) -> (14.8264, 17.8936) centre (8.9451, 20.4371) ccw projected
  arc A564 (14.8264, 17.8936) -> (15.005, 18.3458) centre (7.8625, 20.9058) ccw projected
  arc A565 (15.005, 18.3458) -> (14.7116, 18.6169) centre (0.9435, 3.4284) ccw projected
  arc A566 (14.7116, 18.6169) -> (14.2749, 18.4034) centre (17.8241, 11.6974) ccw projected
  arc A567 (14.2749, 18.4034) -> (13.9325, 18.2085) centre (17.272, 12.7398) ccw projected
  arc A568 (13.9325, 18.2085) -> (13.6702, 18.0374) centre (16.6796, 13.7089) ccw projected
  arc A569 (13.6702, 18.0374) -> (13.3818, 18.2837) centre (0.9435, 3.4284) ccw projected
  arc A570 (13.3818, 18.2837) -> (13.5097, 18.5696) centre (8.6357, 20.579) ccw projected
  arc A571 (13.5097, 18.5696) -> (13.6486, 18.9383) centre (7.5859, 21.0125) ccw projected
  arc A572 (13.6486, 18.9383) -> (13.7912, 19.403) centre (6.47, 21.3947) ccw projected